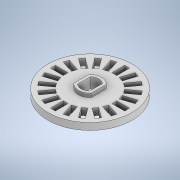
# Autodesk Inventor part: TT encoder disk
Saved by Autodesk Inventor 2022 (Build 260153070, 153G)
## iProperties
Created: 2021-11-27
Part Number: TT encoder disk
Material: Generic
Document SubType Name: Modeling
Designer: a laptop
Density: 1 g/cm^3
Appearance: Default
Author: a laptop
Autodesk Inventor part; units mm, degrees
ref_plane "YZ Plane" through (0, 0, 0) normal (1, 0, 0) x (0, 1, 0)
ref_plane "XZ Plane" through (0, 0, 0) normal (0, 1, 0) x (-1, 0, 0)
ref_plane "XY Plane" through (0, 0, 0) normal (0, 0, 1) x (1, 0, 0)
sketch "Sketch1" plane through (0, 0, 0) normal (0, 1, 0) x (-1, 0, 0)
  circle A0 centre (0, 0) radius 12.875
  arc A1 (-1.85, -1.9666) -> (1.85, -1.9666) centre (0, 0) ccw
  line L0 (1.85, 1.9666) -> (1.85, -1.9666)
  line L1 (-1.85, 1.9666) -> (-1.85, -1.9666)
  line L2 (7.45, 0.75) -> (11.375, 0.75)
  line L3 (11.375, 0.75) -> (11.375, -0.75)
  line L4 (11.375, -0.75) -> (7.45, -0.75)
  line L5 (7.45, -0.75) -> (7.45, 0.75)
  line L6 (0, 0) -> (11.375, 0) construction
  line L7 (11.05, 2.8018) -> (7.3171, 1.5889)
  line L8 (10.5865, 4.2284) -> (11.05, 2.8018)
  line L9 (6.8536, 3.0155) -> (10.5865, 4.2284)
  line L10 (7.3171, 1.5889) -> (6.8536, 3.0155)
  line L11 (9.6434, 6.0793) -> (6.468, 3.7722)
  line L12 (8.7617, 7.2928) -> (9.6434, 6.0793)
  line L13 (5.5863, 4.9858) -> (8.7617, 7.2928)
  line L14 (6.468, 3.7722) -> (5.5863, 4.9858)
  line L15 (7.2928, 8.7617) -> (4.9858, 5.5863)
  line L16 (6.0793, 9.6434) -> (7.2928, 8.7617)
  line L17 (3.7722, 6.468) -> (6.0793, 9.6434)
  line L18 (4.9858, 5.5863) -> (3.7722, 6.468)
  line L19 (4.2284, 10.5865) -> (3.0155, 6.8536)
  line L20 (2.8018, 11.05) -> (4.2284, 10.5865)
  line L21 (1.5889, 7.3171) -> (2.8018, 11.05)
  line L22 (3.0155, 6.8536) -> (1.5889, 7.3171)
  line L23 (0.75, 11.375) -> (0.75, 7.45)
  line L24 (-0.75, 11.375) -> (0.75, 11.375)
  line L25 (-0.75, 7.45) -> (-0.75, 11.375)
  line L26 (0.75, 7.45) -> (-0.75, 7.45)
  line L27 (-2.8018, 11.05) -> (-1.5889, 7.3171)
  line L28 (-4.2284, 10.5865) -> (-2.8018, 11.05)
  line L29 (-3.0155, 6.8536) -> (-4.2284, 10.5865)
  line L30 (-1.5889, 7.3171) -> (-3.0155, 6.8536)
  line L31 (-6.0793, 9.6434) -> (-3.7722, 6.468)
  line L32 (-7.2928, 8.7617) -> (-6.0793, 9.6434)
  line L33 (-4.9858, 5.5863) -> (-7.2928, 8.7617)
  line L34 (-3.7722, 6.468) -> (-4.9858, 5.5863)
  line L35 (-8.7617, 7.2928) -> (-5.5863, 4.9858)
  line L36 (-9.6434, 6.0793) -> (-8.7617, 7.2928)
  line L37 (-6.468, 3.7722) -> (-9.6434, 6.0793)
  line L38 (-5.5863, 4.9858) -> (-6.468, 3.7722)
  line L39 (-10.5865, 4.2284) -> (-6.8536, 3.0155)
  line L40 (-11.05, 2.8018) -> (-10.5865, 4.2284)
  line L41 (-7.3171, 1.5889) -> (-11.05, 2.8018)
  line L42 (-6.8536, 3.0155) -> (-7.3171, 1.5889)
  line L43 (-11.375, 0.75) -> (-7.45, 0.75)
  line L44 (-11.375, -0.75) -> (-11.375, 0.75)
  line L45 (-7.45, -0.75) -> (-11.375, -0.75)
  line L46 (-7.45, 0.75) -> (-7.45, -0.75)
  line L47 (-11.05, -2.8018) -> (-7.3171, -1.5889)
  line L48 (-10.5865, -4.2284) -> (-11.05, -2.8018)
  line L49 (-6.8536, -3.0155) -> (-10.5865, -4.2284)
  line L50 (-7.3171, -1.5889) -> (-6.8536, -3.0155)
  line L51 (-9.6434, -6.0793) -> (-6.468, -3.7722)
  line L52 (-8.7617, -7.2928) -> (-9.6434, -6.0793)
  line L53 (-5.5863, -4.9858) -> (-8.7617, -7.2928)
  line L54 (-6.468, -3.7722) -> (-5.5863, -4.9858)
  line L55 (-7.2928, -8.7617) -> (-4.9858, -5.5863)
  line L56 (-6.0793, -9.6434) -> (-7.2928, -8.7617)
  line L57 (-3.7722, -6.468) -> (-6.0793, -9.6434)
  line L58 (-4.9858, -5.5863) -> (-3.7722, -6.468)
  line L59 (-4.2284, -10.5865) -> (-3.0155, -6.8536)
  line L60 (-2.8018, -11.05) -> (-4.2284, -10.5865)
  line L61 (-1.5889, -7.3171) -> (-2.8018, -11.05)
  line L62 (-3.0155, -6.8536) -> (-1.5889, -7.3171)
  line L63 (-0.75, -11.375) -> (-0.75, -7.45)
  line L64 (0.75, -11.375) -> (-0.75, -11.375)
  line L65 (0.75, -7.45) -> (0.75, -11.375)
  line L66 (-0.75, -7.45) -> (0.75, -7.45)
  line L67 (2.8018, -11.05) -> (1.5889, -7.3171)
  line L68 (4.2284, -10.5865) -> (2.8018, -11.05)
  line L69 (3.0155, -6.8536) -> (4.2284, -10.5865)
  line L70 (1.5889, -7.3171) -> (3.0155, -6.8536)
  line L71 (6.0793, -9.6434) -> (3.7722, -6.468)
  line L72 (7.2928, -8.7617) -> (6.0793, -9.6434)
  line L73 (4.9858, -5.5863) -> (7.2928, -8.7617)
  line L74 (3.7722, -6.468) -> (4.9858, -5.5863)
  line L75 (8.7617, -7.2928) -> (5.5863, -4.9858)
  line L76 (9.6434, -6.0793) -> (8.7617, -7.2928)
  line L77 (6.468, -3.7722) -> (9.6434, -6.0793)
  line L78 (5.5863, -4.9858) -> (6.468, -3.7722)
  line L79 (10.5865, -4.2284) -> (6.8536, -3.0155)
  line L80 (11.05, -2.8018) -> (10.5865, -4.2284)
  line L81 (7.3171, -1.5889) -> (11.05, -2.8018)
  line L82 (6.8536, -3.0155) -> (7.3171, -1.5889)
  arc A2 (-1.85, 1.9666) -> (-1.85, -1.9666) centre (0, 0) ccw construction
  arc A3 (1.85, 1.9666) -> (-1.85, 1.9666) centre (0, 0) ccw
  arc A4 (1.85, -1.9666) -> (1.85, 1.9666) centre (0, 0) ccw construction
  point P0 (10.8183, 3.5151)
  point P1 (9.2026, 6.6861)
  point P2 (6.6861, 9.2026)
  point P3 (3.5151, 10.8183)
  point P4 (0, 11.375)
  point P5 (-3.5151, 10.8183)
  point P6 (-6.6861, 9.2026)
  point P7 (-9.2026, 6.6861)
  point P8 (-10.8183, 3.5151)
  point P9 (-11.375, 0)
  point P10 (-10.8183, -3.5151)
  point P11 (-9.2026, -6.6861)
  point P12 (-6.6861, -9.2026)
  point P13 (-3.5151, -10.8183)
  point P14 (0, -11.375)
  point P15 (3.5151, -10.8183)
  point P16 (6.6861, -9.2026)
  point P17 (9.2026, -6.6861)
  point P18 (10.8183, -3.5151)
  dimension "d0" = 25.75
  dimension "d1" = 5.4
  dimension "d3" = 3.7
  dimension "d4" = 4.75
  dimension "d5" = 1.5
  dimension "d6" = 1.5
  dimension "d9" = 360
  constraints: 166 end point, 9 point on circle, 5 centre point, 4 parallel, 2 coincident, 2 perpendicular, 1 horizontal, 1 midpoint, 1 vertical, 181 other
  measures "d0" diameter of A0
  measures "d1" diameter of A1
  measures "d3" distance between parallel lines of L1 L0
  measures "d4" distance edge to line of A1 L5
  measures "d5" distance edge to line of A0 L3
  measures "d6" distance between parallel lines of L4 L2
extrude "Extrusion1" add sketch "Sketch1" along normal blind 2.1
sketch "Sketch2" plane through (0, 2.1, 0) normal (0, 1, 0) x (1, 0, 0)
  arc A0 (1.85, 1.9666) -> (-1.85, 1.9666) centre (0, 0) ccw projected
  line L0 (1.85, 1.9666) -> (1.85, -1.9666) projected
  arc A1 (-1.85, -1.9666) -> (1.85, -1.9666) centre (0, 0) ccw projected
  line L1 (-1.85, -1.9666) -> (-1.85, 1.9666) projected
  arc A2 (-2.65, -2.2864) -> (2.65, -2.2864) centre (0, 0) ccw
  arc A3 (2.65, 2.2864) -> (-2.65, 2.2864) centre (0, 0) ccw
  line L2 (-2.65, -2.2864) -> (-2.65, 2.2864)
  line L3 (2.65, 2.2864) -> (2.65, -2.2864)
  dimension "d13" = 0.8
  dimension "d14" = 0.8
  dimension "d15" = 0.8
  constraints: 4 end point, 4 point on circle, 3 concentric, 2 centre point, 2 vertical
  measures "d13" distance between parallel lines of L1 L2
  measures "d14" radial gap between concentric circles of A1 A2
  measures "d15" distance between parallel lines of L3 L0
extrude "Extrusion2" add sketch "Sketch2" along normal blind 1.15
body "Solid1"
